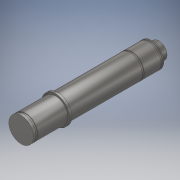
# Autodesk Inventor part: Main Vert Axle
Saved by Autodesk Inventor 2019.4 (Build 234330000, 330)
## iProperties
Created: 2019-11-30
Part Number: Main Vert Axle
Material: Stainless Steel
Document SubType Name: Modeling
Designer: admin
Density: 8 g/cm^3
Appearance: Semi-Polished
Author: admin
Autodesk Inventor part; units mm, degrees
ref_plane "YZ Plane" through (0, 0, 0) normal (1, 0, 0) x (0, 1, 0)
ref_plane "XZ Plane" through (0, 0, 0) normal (0, 1, 0) x (-1, 0, 0)
ref_plane "XY Plane" through (0, 0, 0) normal (0, 0, 1) x (1, 0, 0)
sketch "Sketch1" plane through (0, 0, 0) normal (1, 0, 0) x (0, 1, 0)
  line L0 (0, 0) -> (7.5, 0)
  line L1 (7.5, -20.8) -> (8.5, -20.8)
  line L2 (8.5, -20.8) -> (8.5, -22.3)
  line L3 (8.5, -22.3) -> (7.5, -22.3)
  line L4 (7.5, 0) -> (7.5, -1.5)
  line L5 (7.5, -1.5) -> (7.15, -1.5)
  line L6 (7.15, -1.5) -> (7.15, -2.6)
  line L7 (7.15, -2.6) -> (7.5, -2.6)
  line L8 (7.5, -2.6) -> (7.5, -20.8)
  line L9 (7.5, -22.3) -> (7.5, -66)
  line L10 (7.5, -66) -> (7.15, -66)
  line L11 (7.15, -66) -> (7.15, -67.1)
  line L12 (7.15, -67.1) -> (7.5, -67.1)
  line L13 (7.5, -67.1) -> (7.5, -77.3)
  line L14 (7.5, -77.3) -> (7.15, -77.3)
  line L15 (7.15, -77.3) -> (7.15, -78.4)
  line L16 (7.15, -78.4) -> (7.5, -78.4)
  line L17 (7.5, -78.4) -> (7.5, -79)
  line L18 (7.5, -79) -> (5, -79)
  line L19 (5, -79) -> (5, -83.5)
  line L20 (5, -83.5) -> (0, -83.5)
  line L21 (0, -83.5) -> (0, 0)
  dimension "d0" = 7.5
  dimension "d1" = 8.5
  dimension "d2" = 5
  dimension "d3" = 1.5
  dimension "d4" = 18.2
  dimension "d5" = 1.5
  dimension "d6" = 0.35
  dimension "d7" = 1.1
  dimension "d8" = 0.35
  dimension "d9" = 1.1
  dimension "d10" = 1.1
  dimension "d12" = 44.8
  dimension "d13" = 10.2
  dimension "d14" = 1.7
  dimension "d15" = 4.5
  constraints: 44 end point, 15 perpendicular, 8 point on line, 1 horizontal, 1 vertical
  measures "d0" distance between parallel lines of L21 L8
  measures "d1" distance between parallel lines of L21 L2
  measures "d2" distance between parallel lines of L21 L19
  measures "d3" distance of L0.end L4.end
  measures "d4" distance of L7.end L1.start
  measures "d5" distance of L1.end L2.end
  measures "d6" distance of L6.end L7.end
  measures "d7" distance of L5.end L6.end
  measures "d8" distance of L9.end L10.end
  measures "d9" distance of L10.end L11.end
  measures "d10" distance of L14.end L15.end
  measures "d12" distance between parallel lines of L12 L3
  measures "d13" distance between parallel lines of L14 L12
  measures "d14" distance between parallel lines of L18 L14
  measures "d15" distance of L18.end L19.end
revolve "Revolution1" add sketch "Sketch1" angle 360 about axis through (0, 0, -83.5) along (0, 0, 1)
body "Solid1"
